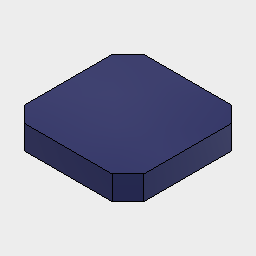
Body (Autodesk Fusion 360 design; units mm, degrees)
Autodesk Fusion 360 part; units mm, degrees
sketch "Sketch1" plane through (0, 0, 0) normal (0, 1, 0) x (1, 0, 0)
  line L0 (30, 30) -> (-30, 30)
  line L1 (-30, 30) -> (-30, -30)
  line L2 (-30, -30) -> (30, -30)
  line L3 (30, -30) -> (30, 30)
  line L4 (30, 30) -> (-30, -30) construction
  line L5 (-30, 30) -> (30, -30) construction
  dimension "d1" = 60
  dimension "d2" = 60
  measures "d1" distance of L0.end L1.end
  measures "d2" distance of L1.end L2.end
extrude "Extrude1" add sketch "Sketch1" along normal blind 12
chamfer "Chamfer1" distance 8 angle 45 1 edges at (30, 6, 30)
chamfer "Chamfer2" distance 8 angle 45 1 edges at (30, 6, -30)
chamfer "Chamfer3" distance 8 angle 45 1 edges at (-30, 6, 30)
chamfer "Chamfer4" distance 8 angle 45 1 edges at (-30, 6, -30)
